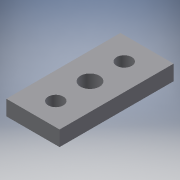
# Autodesk Inventor part: sujetador
Saved by Autodesk Inventor 2018 (Build 220112000, 112)
## iProperties
Created: 2021-07-06
Part Number: sujetador
Material: Genérico
Document SubType Name: Modeling
Designer: GABRIEL
Density: 1 g/cm^3
Appearance: Valor por defecto
Author: GABRIEL
Autodesk Inventor part; units mm, degrees
ref_plane "YZ Plane" through (0, 0, 0) normal (1, 0, 0) x (0, 1, 0)
ref_plane "XZ Plane" through (0, 0, 0) normal (0, 1, 0) x (-1, 0, 0)
ref_plane "XY Plane" through (0, 0, 0) normal (0, 0, 1) x (1, 0, 0)
sketch "Boceto1" plane through (0, 0, 0) normal (0, 0, 1) x (1, 0, 0)
  line L0 (0, 0) -> (70, 0)
  line L1 (70, 0) -> (70, -150)
  line L2 (70, -150) -> (0, -150)
  line L3 (0, -150) -> (0, 0)
  circle A0 centre (35, -30) radius 10
  circle A1 centre (35, -120) radius 10
  circle A2 centre (35, -75) radius 12.5
  dimension "d0" = 70
  dimension "d1" = 150
  dimension "d2" = 20
  dimension "d3" = 20
  dimension "d4" = 25
  dimension "d5" = 35
  dimension "d6" = 30
  dimension "d7" = 35
  dimension "d8" = 75
  dimension "d9" = 35
  dimension "d10" = 120
  constraints: 8 end point, 3 centre point, 2 parallel, 1 horizontal, 1 perpendicular
  measures "d0" distance of L1.end L2.end
  measures "d1" distance of L0.end L1.end
  measures "d2" diameter of A0
  measures "d3" diameter of A1
  measures "d4" diameter of A2
  measures "d5" distance from line of A0.centre L1
  measures "d6" distance from line of A0.centre L0
  measures "d7" distance from line of A2.centre L1
  measures "d8" distance from line of A2.centre L0
  measures "d9" distance from line of A1.centre L1
  measures "d10" distance from line of A1.centre L0
extrude "Extrusión1" add sketch "Boceto1" along normal blind 20
